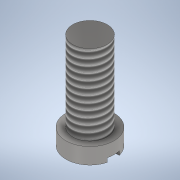
# Autodesk Inventor part: Screw_Terminal
Saved by Autodesk Inventor 2020 (Build 240168000, 168)
## iProperties
Created: 2019-08-19
Part Number: Screw_Terminal
Material: Generic
Document SubType Name: Modeling
Designer: SENSE IT OUT
Density: 1 g/cm^3
Appearance: Default
Author: SENSE IT OUT
Autodesk Inventor part; units mm, degrees
ref_plane "YZ Plane" through (0, 0, 0) normal (1, 0, 0) x (0, 1, 0)
ref_plane "XZ Plane" through (0, 0, 0) normal (0, 1, 0) x (-1, 0, 0)
ref_plane "XY Plane" through (0, 0, 0) normal (0, 0, 1) x (1, 0, 0)
sketch "Sketch1" plane through (0, 0, 0) normal (0, 1, 0) x (-1, 0, 0)
  circle A0 centre (0, 0) radius 1.5
  dimension "d0" = 3
  constraints: 1 centre point, 1 coincident
  measures "d0" diameter of A0
extrude "Extrusion1" add sketch "Sketch1" along normal blind 1
sketch "Sketch2" plane through (0, 1, 0) normal (0, 1, 0) x (1, 0, 0)
  circle A0 centre (0, 0) radius 1.078
  dimension "d3" = 2.156
  constraints: 1 centre point, 1 coincident
  measures "d3" diameter of A0
extrude "Extrusion2" add sketch "Sketch2" along normal blind 5
thread "Thread1" size "M2x0.4" class "6g" standard "ANSI Metric M Profile" full length
sketch "Sketch3" plane through (0, 0, 0) normal (0, -1, 0) x (1, 0, 0)
  line L0 (1.6528, 0.375) -> (-2.2622, 0.375)
  line L1 (-2.2622, 0.375) -> (-2.2622, -0.375)
  line L2 (-2.2622, -0.375) -> (1.6528, -0.375)
  line L3 (1.6528, -0.375) -> (1.6528, 0.375)
  point P0 (0, 0)
  dimension "d8" = 0.75
  dimension "d9" = 0.375
  constraints: 8 end point, 2 parallel, 1 horizontal, 1 perpendicular
  measures "d8" distance between parallel lines of L0 L2
  measures "d9" distance from line of point (0, 0) L2
extrude "Extrusion3" cut sketch "Sketch3" against normal blind 0.25
body "Solid1"
